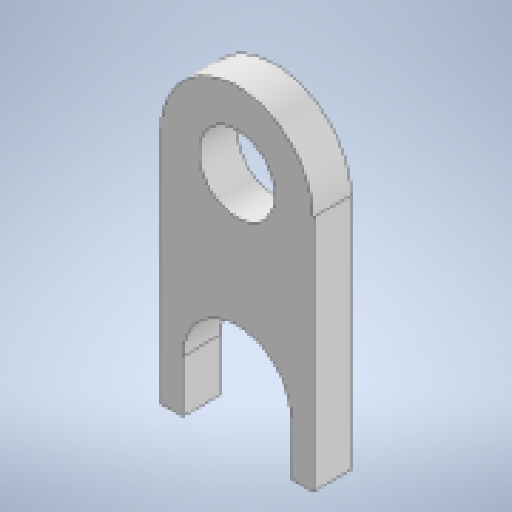
# Autodesk Inventor part: display-retainer-tab
Saved by Autodesk Inventor 2024 (Build 280153000, 153)
## iProperties
Created: 2024-08-25
Part Number: display-retainer-tab
Material: Generic
Document SubType Name: Modeling
Designer: Stefano
Density: 1 g/cm^3
Appearance: Default
Author: Stefano
Autodesk Inventor part; units mm, degrees
ref_plane "YZ Plane" through (0, 0, 0) normal (1, 0, 0) x (0, 1, 0)
ref_plane "XZ Plane" through (0, 0, 0) normal (0, 1, 0) x (-1, 0, 0)
ref_plane "XY Plane" through (0, 0, 0) normal (0, 0, 1) x (1, 0, 0)
sketch "Sketch1" plane through (0, 0, 0) normal (0, 0, 1) x (1, 0, 0)
  circle A0 centre (0, 5) radius 1.5 construction
  circle A1 centre (0, -4.7587) radius 2.75 construction
  circle A2 centre (0, 5) radius 4
  line L0 (4, -7.5087) -> (-4, -7.5087)
  line L1 (-4, -7.5087) -> (-4, 5)
  line L2 (4, -7.5087) -> (4, 5)
  circle A3 centre (0, -4.7587) radius 2.85
  line L3 (2.85, -4.7587) -> (2.85, -7.5087)
  line L4 (-2.85, -4.7587) -> (-2.85, -7.5087)
  circle A4 centre (0, 5) radius 2
  point P0 (0, 0)
  dimension "d0" = 8
  dimension "d1" = 0.1
  dimension "d2" = 4
  constraints: 10 end point, 5 tangent, 4 point on circle, 3 centre point, 2 coincident, 2 parallel, 2 perpendicular, 2 point on line, 1 horizontal
  measures "d0" diameter of A2
  measures "d1" radial gap between concentric circles of A1 A3
  measures "d2" diameter of A4
extrude "Extrusion1" add sketch "Sketch1" along normal blind 2 contours A2 | L2 L0 L3 A3 L4 L1 A2
sketch "Sketch3" plane through (0, 0, 2) normal (0, 0, 1) x (1, 0, 0)
  line L0 (-4, 5) -> (-4, -7.5087) projected
  line L1 (-4, -7.5087) -> (-2.85, -7.5087) projected
  line L2 (-2.85, -7.5087) -> (-2.85, -4.7587) projected
  arc A0 (2.85, -4.7587) -> (-2.85, -4.7587) centre (0, -4.7587) ccw projected
  line L3 (2.85, -4.7587) -> (2.85, -7.5087) projected
  line L4 (2.85, -7.5087) -> (4, -7.5087) projected
  line L5 (4, -7.5087) -> (4, 5) projected
  arc A1 (4, 5) -> (-4, 5) centre (0, 5) ccw projected
  circle A2 centre (0, 5) radius 2 projected
  circle A3 centre (0, 5) radius 2 construction
  line L6 (0, 3) -> (0, -1.9087) construction
  line L7 (4, -7.5087) -> (4, 5) projected
  line L8 (4, 0.5456) -> (-4, 0.5456)
  arc A4 (2.85, -4.7587) -> (-2.85, -4.7587) centre (0, -4.7587) ccw projected
  point P0 (0, 0)
  point P1 (0, 0.5456)
  point P2 (0, -1.9087)
  constraints: 4 end point, 3 point on line, 2 midpoint, 2 point on circle, 1 perpendicular, 1 vertical alignment, 1 other
extrude "Extrusion2" add sketch "Sketch3" along normal blind 1 contours L8 L5 L4 L3 A0 L2 L1 L0
chamfer "Chamfer1" distance 1 angle 45 1 edges at (0, 0.5456, 3)
body "Solid1"
